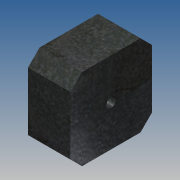
# Autodesk Inventor part: Mittelteil
Saved by Autodesk Inventor 2015 (Build 190159000, 159)
## iProperties
Created: 2015-01-06
Part Number: Mittelteil
Material: Stahl
Document SubType Name: Modeling
Designer: Marc
Mass: 399.798 g
Surface Area: 85.2078 cm^2
Volume: 50.9297 cm^3
Density: 7.85 g/cm^3
Appearance: Platte
Author: Marc
Autodesk Inventor part; units mm, degrees
ref_plane "YZ Plane" through (0, 0, 0) normal (1, 0, 0) x (0, 1, 0)
ref_plane "XZ Plane" through (0, 0, 0) normal (0, 1, 0) x (-1, 0, 0)
ref_plane "XY Plane" through (0, 0, 0) normal (0, 0, 1) x (1, 0, 0)
sketch "Skizze1" plane through (0, 0, 0) normal (1, 0, 0) x (0, 1, 0)
  line L0 (-29.61, 0) -> (29.61, 0) projected
  line L1 (0, -29.61) -> (0, 29.61) projected
  line L2 (-15.15, 21.15) -> (15.15, 21.15)
  line L3 (21.15, 15.15) -> (21.15, -15.15)
  line L4 (15.15, -21.15) -> (-15.15, -21.15)
  line L5 (-21.15, -15.15) -> (-21.15, 15.15)
  line L6 (15.15, 21.15) -> (21.15, 15.15)
  line L7 (21.15, -15.15) -> (15.15, -21.15)
  line L8 (-15.15, -21.15) -> (-21.15, -15.15)
  line L9 (-15.15, 21.15) -> (-21.15, 15.15)
  circle A0 centre (0, 0) radius 2.5
  point P0 (-21.15, 21.15)
  point P1 (21.15, -21.15)
  point P2 (21.15, 21.15)
  point P3 (-21.15, -21.15)
  dimension "d0" = 42.3
  dimension "d1" = 42.3
  dimension "d2" = 6
  dimension "d3" = 6
  dimension "d4" = 6
  dimension "d5" = 6
  dimension "d6" = 6
  dimension "d7" = 6
  dimension "d8" = 6
  dimension "d9" = 6
  dimension "d10" = 5
  constraints: 16 end point, 8 point on line, 2 parallel, 1 centre point, 1 coincident, 1 horizontal, 1 perpendicular, 2 other
  measures "d0" distance of point (21.15, -21.15) point (-21.15, -21.15)
  measures "d1" distance of point (21.15, 21.15) point (21.15, -21.15)
  measures "d2" distance of L2.end point (21.15, 21.15)
  measures "d3" distance of L3.start point (21.15, 21.15)
  measures "d4" distance of L3.end point (21.15, -21.15)
  measures "d5" distance of L4.start point (21.15, -21.15)
  measures "d6" distance of L4.end point (-21.15, -21.15)
  measures "d7" distance of L5.start point (-21.15, -21.15)
  measures "d8" distance of L2.start point (-21.15, 21.15)
  measures "d9" distance of L5.end point (-21.15, 21.15)
  measures "d10" diameter of A0
extrude "Extrusion1" add sketch "Skizze1" along normal mid plane 22 contours L5 L9 L2 L1 A0 L0 | L0 A0 L1 L4 L8 L5 | L1 L2 L6 L3 L0 A0 | A0 L0 L3 L7 L4 L1
equation "\"d3\" = d2"
equation "\"d4\" = d2"
equation "\"d5\" = d4"
equation "\"d6\" = d2"
equation "\"d7\" = d6"
equation "\"d8\" = d2"
equation "\"d9\" = d8"
